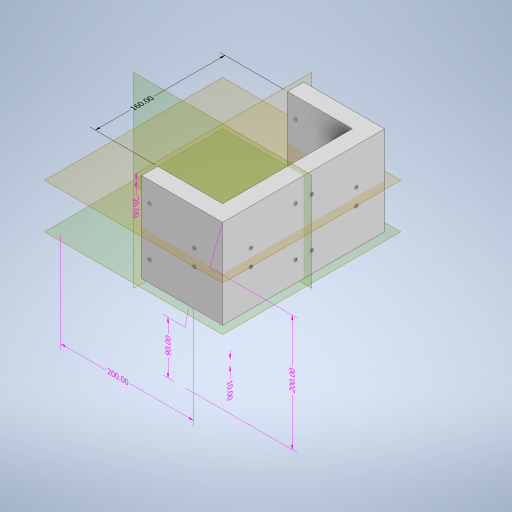
# Autodesk Inventor part: container_front_head_1
Saved by Autodesk Inventor 2023 (Build 270158000, 158)
## iProperties
Created: 2022-10-30
Part Number: container_front_head_1
Material: Genérico
Document SubType Name: Modeling
Designer: papel
Density: 1 g/cm^3
Appearance: Valor por defecto
Surface Area: 1558.19 cm^2
Author: papel
Autodesk Inventor part; units mm, degrees
ref_plane "YZ Plane" through (0, 0, 0) normal (1, 0, 0) x (0, 1, 0)
ref_plane "XZ Plane" through (0, 0, 0) normal (0, 1, 0) x (-1, 0, 0)
ref_plane "XY Plane" through (0, 0, 0) normal (0, 0, 1) x (1, 0, 0)
sketch "Boceto2" plane through (0, 0, 0) normal (0, 1, 0) x (-1, 0, 0)
  line L0 (7.5, 100) -> (-7.5, 100)
  line L1 (-7.5, 100) -> (-7.5, -100)
  line L2 (-7.5, -100) -> (7.5, -100)
  line L3 (7.5, -100) -> (7.5, 100)
  line L4 (7.5, 100) -> (-7.5, -100) construction
  line L5 (-7.5, 100) -> (7.5, -100) construction
  point P0 (0, 0)
  dimension "d7" = 15
  dimension "d8" = 200
  constraints: 12 end point, 2 midpoint, 2 parallel, 1 horizontal, 1 perpendicular
  measures "d7" distance of L2.end L1.end
  measures "d8" distance of L1.end L0.end
extrude "Extrusión1" add sketch "Boceto2" along normal blind 10
sketch "Boceto3" plane through (0, 10, 0) normal (0, 1, 0) x (1, 0, 0)
  circle A0 centre (3.25, 58.25) radius 1.75
  line L0 (5, 50) -> (-5, 50)
  line L1 (-5, 50) -> (-5, 60)
  line L2 (-5, 60) -> (5, 60)
  line L3 (5, 60) -> (5, 50)
  line L4 (5, 50) -> (-5, 60) construction
  line L5 (-5, 50) -> (5, 60) construction
  circle A1 centre (-3.25, 51.75) radius 1.75
  line L6 (7.5, 100) -> (-7.5, 100) projected
  line L7 (-7.5, 0) -> (3.408, 0)
  line L8 (5, -60) -> (5, -50)
  line L9 (-5, -60) -> (5, -60)
  line L10 (5, -50) -> (-5, -50)
  line L11 (-5, -50) -> (-5, -60)
  line L12 (-5, -50) -> (5, -60) construction
  circle A2 centre (-3.25, -51.75) radius 1.75
  line L13 (5, -50) -> (-5, -60) construction
  circle A3 centre (3.25, -58.25) radius 1.75
  line L14 (-7.5, -100) -> (7.5, -100) projected
  point P0 (0, 0)
  point P1 (-5, 55)
  point P2 (0, 100)
  point P3 (-5, -55)
  dimension "d11" = 3.5
  dimension "d12" = 1.75
  dimension "d13" = 1.75
  dimension "d14" = 1.75
  dimension "d15" = 1.75
  dimension "d16" = 10
  dimension "d17" = 10
  dimension "d19" = 40
  dimension "d81" = 40
  constraints: 26 end point, 7 symmetric about line, 4 centre point, 2 horizontal, 2 midpoint, 2 parallel, 1 perpendicular, 2 other
  measures "d11" diameter of A0
  measures "d12" distance from line of L2 A0.centre
  measures "d13" distance from line of L3 A0.centre
  measures "d14" distance from line of L1 A1.centre
  measures "d15" distance from line of L0 A1.centre
  measures "d16" distance between parallel lines of L0 L2
  measures "d17" distance between parallel lines of L3 L1
  measures "d19" distance from line of point (0, 100) L2
  measures "d81" distance between parallel lines of L14 L9
hole "Agujero1" at (3.25, 10, 58.25) at (-3.25, 10, 51.75) at (3.25, 10, -58.25) at (-3.25, 10, -51.75) direction (0, -1, 0) diameter 3.5 end through all
sketch "Boceto4" plane through (0, 10, 0) normal (0, 1, 0) x (1, 0, 0)
  line L0 (-7.5, 100) -> (-7.5, -100) projected
  line L1 (-7.5, -100) -> (7.5, -100)
  line L2 (7.5, -100) -> (7.5, -80)
  line L3 (7.5, -80) -> (-7.5, -80)
  line L4 (-7.5, -80) -> (-7.5, -100)
  line L5 (-7.5, 0) -> (1.0116, 0)
  line L6 (-7.5, -100) -> (-7.5, 100)
  line L7 (-7.5, 100) -> (7.5, 100)
  line L8 (7.5, 100) -> (7.5, 80)
  line L9 (7.5, 80) -> (-7.5, 80)
  line L10 (-7.5, 80) -> (-7.5, 100)
  point P0 (0, 0)
  point P1 (-7.5, -80)
  point P2 (-7.5, 80)
  dimension "d27" = 15
  dimension "d28" = 20
  constraints: 20 end point, 5 symmetric about line, 2 horizontal, 2 parallel, 1 midpoint, 1 perpendicular
  measures "d27" distance of L3.end L2.end
  measures "d28" distance of L2.end L1.end
extrude "Extrusión2" add sketch "Boceto4" along normal blind 80
sketch "Boceto5" plane through (0, 90, 0) normal (0, 1, 0) x (1, 0, 0)
  line L0 (-7.5, -100) -> (7.5, -100) projected
  line L1 (-7.5, -100) -> (49.5, -100)
  line L2 (49.5, -100) -> (49.5, 100)
  line L3 (49.5, 100) -> (-7.5, 100)
  line L4 (-7.5, 100) -> (-7.5, -100)
  line L5 (49.5, -100) -> (-150.5, -100)
  line L6 (-150.5, -100) -> (-150.5, 100)
  line L7 (-150.5, 100) -> (49.5, 100)
  line L8 (49.5, 100) -> (49.5, -100)
  point P0 (0, 0)
  point P1 (-7.5, 100)
  dimension "d31" = 57
  dimension "d32" = 200
  dimension "d75" = 200
  constraints: 16 end point, 4 parallel, 2 horizontal, 2 perpendicular, 1 point on line
  measures "d31" distance of L3.end L2.end
  measures "d32" distance of L6.end L7.end
  measures "d75" distance between parallel lines of L5 L7
extrude "Extrusión3" add sketch "Boceto5" along normal blind 110
sketch "Boceto6" plane through (0, 200, 0) normal (0, 1, 0) x (1, 0, 0)
  line L0 (49.5, 100) -> (7.5, 100) projected
  line L1 (49.5, 100) -> (29.5, 100)
  line L2 (29.5, 100) -> (29.5, 80)
  line L3 (7.5, -100) -> (49.5, -100) projected
  line L4 (28.5, -100) -> (28.5, -80)
  line L5 (-150.5, 100) -> (-150.5, -100) projected
  line L6 (29.5, 80) -> (-150.5, 80)
  line L7 (-150.5, 80) -> (-150.5, -80)
  line L8 (-150.5, -80) -> (29.5, -80)
  line L9 (29.5, -80) -> (29.5, 80)
  line L10 (-150.5, -100) -> (49.5, -100) projected
  point P0 (7.5, 80)
  point P1 (-50.5, -100)
  dimension "d36" = 20
  dimension "d37" = 20
  dimension "d38" = 20
  dimension "d77" = 20
  constraints: 14 end point, 2 midpoint, 2 parallel, 2 perpendicular, 2 point on line, 1 horizontal, 1 vertical
  measures "d36" distance of L0.start L1.end
  measures "d37" distance of L1.end L2.end
  measures "d38" distance of L4.start L4.end
  measures "d77" distance from line of point (-50.5, -100) L8
extrude "Extrusión4" cut sketch "Boceto6" against normal blind 90 contours L8 L5 L6 L9
sketch "Boceto7" plane through (-150.5, 90, -100) normal (-1, 0, 0) x (0, 0, 1)
  line L0 (0, 110) -> (20, 110) projected
  line L1 (20, 110) -> (10, 110)
  line L2 (10, 110) -> (10, 20)
  line L3 (10, 20) -> (20, 20)
  line L4 (20, 20) -> (20, 110)
  line L5 (180, 110) -> (180, 20) projected
  line L6 (180, 110) -> (190, 110)
  line L7 (190, 110) -> (190, 20)
  line L8 (190, 20) -> (180, 20)
  line L9 (180, 20) -> (180, 110)
  line L10 (200, 0) -> (200, 110) projected
  line L11 (0, 0) -> (0, 110) projected
  line L12 (0, 110) -> (10, 110)
  line L13 (10, 110) -> (10, 20)
  line L14 (10, 20) -> (0, 20)
  line L15 (0, 20) -> (0, 110)
  line L16 (200, 110) -> (0, 110) projected
  line L17 (200, 110) -> (190, 110)
  line L18 (190, 110) -> (190, 20)
  line L19 (190, 20) -> (200, 20)
  line L20 (200, 20) -> (200, 110)
  point P0 (100, -90)
  dimension "d63" = 10
  dimension "d65" = 10
  dimension "d76" = 10
  constraints: 32 end point, 8 parallel, 4 horizontal, 4 perpendicular, 1 point on line
  measures "d63" distance between parallel lines of L10 L7
  measures "d65" distance between parallel lines of L11 L2
  measures "d76" distance between parallel lines of L20 L7
extrude "Extrusión5" cut sketch "Boceto7" against normal blind 30 contours L0 L4 L3 L2 | L6 L7 L8 L5
sketch "Boceto8" plane through (-7.5, 0, 100) normal (0, 0, 1) x (1, 0, 0)
  line L0 (-113, 110) -> (-113, 200) projected
  line L1 (-113, 200) -> (-113, 110)
  circle A0 centre (-124.75, 183.25) radius 1.75
  line L2 (-123, 175) -> (-133, 175)
  line L3 (-133, 175) -> (-133, 185)
  line L4 (-133, 185) -> (-123, 185)
  line L5 (-123, 185) -> (-123, 175)
  line L6 (-123, 175) -> (-133, 185) construction
  line L7 (-133, 175) -> (-123, 185) construction
  circle A1 centre (-131.25, 176.75) radius 1.75
  line L8 (-143, 200) -> (57, 200) projected
  line L9 (-143, 90) -> (-143, 200) projected
  line L10 (-113, 155) -> (-128, 155)
  line L11 (-123, 125) -> (-123, 135)
  line L12 (-133, 125) -> (-123, 125)
  line L13 (-123, 135) -> (-133, 125) construction
  line L14 (-123, 135) -> (-133, 135)
  line L15 (-133, 135) -> (-123, 125) construction
  circle A2 centre (-131.25, 133.25) radius 1.75
  line L16 (-133, 135) -> (-133, 125)
  circle A3 centre (-124.75, 126.75) radius 1.75
  line L17 (-143, 110) -> (-113, 110) projected
  point P0 (7.5, 0)
  point P1 (-133, 180)
  point P2 (-123, 180)
  point P3 (-133, 130)
  point P4 (-123, 130)
  dimension "d45" = 3.5
  dimension "d46" = 1.75
  dimension "d47" = 1.75
  dimension "d48" = 1.75
  dimension "d49" = 1.75
  dimension "d50" = 10
  dimension "d51" = 10
  dimension "d52" = 15
  dimension "d53" = 10
  dimension "d54" = 10
  dimension "d55" = 15
  constraints: 28 end point, 8 symmetric about line, 4 centre point, 3 equal length, 3 midpoint, 2 horizontal, 1 perpendicular, 2 other
  measures "d45" diameter of A0
  measures "d46" distance from line of L4 A0.centre
  measures "d47" distance from line of L5 A0.centre
  measures "d48" distance from line of L3 A1.centre
  measures "d49" distance from line of L2 A1.centre
  measures "d50" distance between parallel lines of L2 L4
  measures "d51" distance between parallel lines of L5 L3
  measures "d52" distance between parallel lines of L8 L4
  measures "d53" distance between parallel lines of L9 L3
  measures "d54" distance from line of L0 point (-123, 180)
  measures "d55" distance between parallel lines of L17 L12
hole "Agujero2" at (-132.25, 183.25, 100) at (-138.75, 176.75, 100) at (-138.75, 133.25, 100) at (-132.25, 126.75, 100) direction (0, 0, -1) diameter 3.5 end through all
ref_plane "Plano de trabajo1" through (-150.5, 90, 100) normal (0, -1, 0) x (1, 0, 0)
split "Dividir1" plane through (-150.5, 90, 100) removes the side toward (0, -1, 0)
ref_plane "Plano de trabajo2" through (49.5, 90, 0) normal (0, 0, -1) x (-1, 0, 0)
ref_plane "Plano de trabajo3" through (-50.5, 90, 100) normal (1, 0, 0) x (0, 0, -1)
ref_plane "Plano de trabajo4" through (0, 145, 0) normal (0, 1, 0) x (1, 0, 0)
sketch "Boceto9" plane through (-150.5, 90, 100) normal (0, 0, 1) x (1, 0, 0)
  line L0 (85.0357, 30) -> (115.0357, 30)
  circle A0 centre (110.0357, 25) radius 1.75
  line L1 (90.0357, 25) -> (110.0357, 25)
  line L2 (115.0357, 30) -> (115.0357, 20)
  circle A1 centre (90.0357, 25) radius 1.75
  line L3 (85.0357, 20) -> (115.0357, 30) construction
  line L4 (85.0357, 30) -> (115.0357, 20) construction
  line L5 (85.0357, 20) -> (85.0357, 30)
  line L6 (115.0357, 20) -> (85.0357, 20)
  line L7 (200, 0) -> (200, 110)
  line L8 (200, 55) -> (88.2857, 55)
  circle A2 centre (90.0357, 85) radius 1.75
  line L9 (85.0357, 80) -> (115.0357, 80)
  line L10 (85.0357, 80) -> (115.0357, 90) construction
  line L11 (85.0357, 90) -> (85.0357, 80)
  line L12 (115.0357, 90) -> (85.0357, 90)
  line L13 (85.0357, 90) -> (115.0357, 80) construction
  circle A3 centre (110.0357, 85) radius 1.75
  line L14 (90.0357, 85) -> (110.0357, 85)
  line L15 (115.0357, 80) -> (115.0357, 90)
  line L16 (100.0357, 55) -> (185.099, 55) construction
  line L17 (160, 70) -> (160, 40)
  circle A4 centre (165, 45) radius 1.75
  line L18 (170, 40) -> (170, 70)
  line L19 (170, 70) -> (160, 40) construction
  line L20 (160, 40) -> (170, 40)
  line L21 (160, 70) -> (170, 40) construction
  circle A5 centre (165, 65) radius 1.75
  line L22 (165, 65) -> (165, 45)
  line L23 (170, 70) -> (160, 70)
  circle A6 centre (55, 65) radius 1.75
  line L24 (60, 70) -> (60, 40)
  line L25 (60, 40) -> (50, 40)
  circle A7 centre (55, 45) radius 1.75
  line L26 (55, 65) -> (55, 45)
  line L27 (60, 70) -> (50, 40) construction
  line L28 (50, 40) -> (50, 70)
  line L29 (50, 70) -> (60, 40) construction
  line L30 (50, 70) -> (60, 70)
  line L31 (30, 110) -> (30, 20)
  point P0 (150.5, -90)
  point P1 (100.0357, 34.7141)
  point P2 (100.0357, 34.7141)
  point P3 (85.0357, 36.6749)
  point P4 (115.0357, 25)
  point P5 (115.0357, 85)
  point P6 (189.1833, 40)
  point P7 (165, 70)
  point P8 (70.0357, 40)
  point P9 (55, 70)
  dimension "d89" = 10
  dimension "d90" = 30
  dimension "d91" = 5
  dimension "d92" = 5
  dimension "d93" = 5
  dimension "d94" = 5
  dimension "d95" = 30
  dimension "d96" = 5
  dimension "d97" = 5
  dimension "d98" = 3.5
  dimension "d99" = 5
  dimension "d100" = 5
  dimension "d101" = 5
  dimension "d102" = 5
  dimension "d103" = 5
  dimension "d104" = 20
  constraints: 58 end point, 8 centre point, 7 symmetric about line, 4 midpoint, 2 horizontal, 1 point on line, 11 other
  measures "d89" distance between parallel lines of L6 L0
  measures "d90" distance between parallel lines of L5 L2
  measures "d91" distance of point (115.036, 25) A0.centre
  measures "d92" distance from line of L0 A0.centre
  measures "d93" distance from line of L0 A1.centre
  measures "d94" distance from line of L5 A1.centre
  measures "d95" distance between parallel lines of L7 L18
  measures "d96" distance from line of L17 L22.start
  measures "d97" distance of point (165, 70) L22.start
  measures "d98" diameter of A4
  measures "d99" distance from line of L20 L22.end
  measures "d100" distance from line of L17 L22.end
  measures "d101" distance of point (55, 70) L26.start
  measures "d102" distance from line of L24 L26.end
  measures "d103" distance from line of L25 L26.end
  measures "d104" distance between parallel lines of L31 L28
hole "Agujero3" at (-60.4643, 175, 100) at (-40.4643, 175, 100) at (14.5, 155, 100) at (-95.5, 155, 100) at (-95.5, 135, 100) at (-60.4643, 115, 100) at (-40.4643, 115, 100) at (14.5, 135, 100) direction (0, 0, -1) diameter 3.5 end through all
sketch "Boceto10" plane through (49.5, 90, 100) normal (1, 0, 0) x (0, 0, -1)
  line L0 (85.0357, 30) -> (115.0357, 30)
  circle A0 centre (110.0357, 25) radius 1.75
  line L1 (90.0357, 25) -> (110.0357, 25)
  line L2 (115.0357, 30) -> (115.0357, 20)
  circle A1 centre (90.0357, 25) radius 1.75
  line L3 (85.0357, 30) -> (115.0357, 20) construction
  line L4 (85.0357, 20) -> (85.0357, 30)
  line L5 (115.0357, 20) -> (85.0357, 20)
  line L6 (85.0357, 20) -> (115.0357, 30) construction
  line L7 (160, 70) -> (160, 40)
  circle A2 centre (165, 45) radius 1.75
  line L8 (160, 40) -> (170, 40)
  line L9 (165, 65) -> (165, 45)
  circle A3 centre (165, 65) radius 1.75
  line L10 (170, 70) -> (160, 40) construction
  line L11 (170, 70) -> (160, 70)
  line L12 (160, 70) -> (170, 40) construction
  line L13 (170, 40) -> (170, 70)
  line L14 (40, 70) -> (40, 40)
  line L15 (35, 65) -> (35, 45)
  circle A4 centre (35, 65) radius 1.75
  line L16 (40, 40) -> (30, 40)
  line L17 (40, 70) -> (30, 40) construction
  line L18 (30, 70) -> (40, 40) construction
  line L19 (30, 70) -> (40, 70)
  line L20 (30, 40) -> (30, 70)
  circle A5 centre (35, 45) radius 1.75
  circle A6 centre (90.0357, 85) radius 1.75
  line L21 (85.0357, 80) -> (115.0357, 80)
  line L22 (115.0357, 80) -> (115.0357, 90)
  circle A7 centre (110.0357, 85) radius 1.75
  line L23 (90.0357, 85) -> (110.0357, 85)
  line L24 (85.0357, 80) -> (115.0357, 90) construction
  line L25 (85.0357, 90) -> (85.0357, 80)
  line L26 (115.0357, 90) -> (85.0357, 90)
  line L27 (85.0357, 90) -> (115.0357, 80) construction
  line L28 (0, 0) -> (0, 110)
  line L29 (200, 0) -> (200, 110)
  point P0 (100, -90)
  point P1 (100.0357, 34.7141)
  point P2 (100.0357, 34.7141)
  point P3 (85.0357, 36.6749)
  point P4 (115.0357, 25)
  point P5 (88.2857, 55)
  point P6 (189.1833, 40)
  point P7 (165, 70)
  point P8 (70.0357, 40)
  point P9 (35, 70)
  point P10 (115.0357, 85)
  point P11 (100.0357, 55)
  dimension "d112" = 10
  dimension "d113" = 30
  dimension "d114" = 5
  dimension "d115" = 5
  dimension "d116" = 5
  dimension "d117" = 5
  dimension "d118" = 5
  dimension "d119" = 5
  dimension "d120" = 3.5
  dimension "d121" = 5
  dimension "d122" = 5
  dimension "d123" = 5
  dimension "d124" = 5
  dimension "d125" = 5
  dimension "d126" = 30
  dimension "d127" = 30
  constraints: 54 end point, 8 centre point, 3 midpoint, 9 other
  measures "d112" distance between parallel lines of L5 L0
  measures "d113" distance between parallel lines of L4 L2
  measures "d114" distance of point (115.036, 25) A0.centre
  measures "d115" distance from line of L0 A0.centre
  measures "d116" distance from line of L0 A1.centre
  measures "d117" distance from line of L4 A1.centre
  measures "d118" distance from line of L7 L9.start
  measures "d119" distance of point (165, 70) L9.start
  measures "d120" diameter of A2
  measures "d121" distance from line of L8 L9.end
  measures "d122" distance from line of L7 L9.end
  measures "d123" distance of point (35, 70) L15.start
  measures "d124" distance from line of L14 L15.end
  measures "d125" distance from line of L16 L15.end
  measures "d126" distance between parallel lines of L28 L20
  measures "d127" distance between parallel lines of L29 L13
hole "Agujero4" at (49.5, 175, 9.9643) at (49.5, 175, -10.0357) at (49.5, 155, 65) at (49.5, 135, 65) at (49.5, 115, 9.9643) at (49.5, 115, -10.0357) at (49.5, 135, -65) at (49.5, 155, -65) direction (-1, 0, 0) diameter 3.5 end through all
split "Dividir2" plane through (-50.5, 90, 100) removes the side toward (-1, 0, 0)
